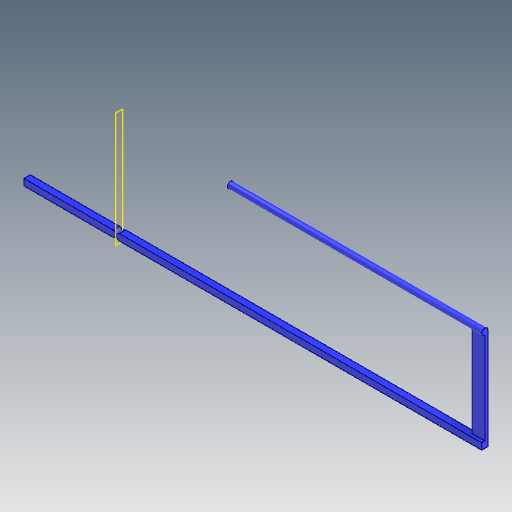
# Autodesk Inventor part: Bone_16_10_Fix
Saved by Autodesk Inventor 2020 (Build 240168000, 168)
## iProperties
Created: 2021-03-17
Part Number: Bone_16_10_Fix
Material: Generic
Document SubType Name: Modeling
Designer: deox
Density: 1 g/cm^3
Appearance: Blue - Wall Paint - Glossy
Author: deox
Autodesk Inventor part; units mm, degrees
ref_plane "YZ Plane" through (0, 0, 0) normal (1, 0, 0) x (0, 1, 0)
ref_plane "XZ Plane" through (0, 0, 0) normal (0, 1, 0) x (-1, 0, 0)
ref_plane "XY Plane" through (0, 0, 0) normal (0, 0, 1) x (1, 0, 0)
sketch "Sketch1" plane through (0, 0, 0) normal (1, 0, 0) x (0, 1, 0)
  circle A0 centre (0, 0) radius 0.05
  line L0 (0, 0) -> (-1.539, 0)
  line L1 (-1.589, 0.05) -> (-1.489, 0.05)
  line L2 (-1.489, 0.05) -> (-1.489, -0.05)
  line L3 (-1.489, -0.05) -> (-1.589, -0.05)
  line L4 (-1.589, -0.05) -> (-1.589, 0.05)
  line L5 (-1.589, 0.05) -> (-1.489, -0.05) construction
  line L6 (-1.489, 0.05) -> (-1.589, -0.05) construction
  line L7 (-1.489, -0.05) -> (0, -0.05)
  point P0 (-0.05, 0)
  point P1 (-1.489, 0)
  dimension "d0" = 0.1
  dimension "d1" = 1.539
  dimension "d2" = 0.1
  dimension "d3" = 0.1
  constraints: 16 end point, 2 horizontal, 2 midpoint, 2 parallel, 1 coincident, 1 perpendicular, 1 point on line, 3 other
  measures "d1" distance of L0.start L0.end
  measures "d2" distance of L2.end L3.end
  measures "d3" distance of L1.end L2.end
extrude "Extrusion1" add sketch "Sketch1" along normal blind 0.2
sketch "Sketch2" plane through (0, 0, 0) normal (-1, 0, 0) x (0, 0, 1)
  arc A0 (0, -0.05) -> (-0.05, 0) centre (0, 0) ccw projected
  circle A1 centre (0, 0) radius 0.05
  point P0 (-0.05, 0)
  point P1 (0, -0.05)
  dimension "d6" = 0.1
  constraints: 1 centre point, 1 coincident
  measures "d6" diameter of A1
extrude "Extrusion2" add sketch "Sketch2" along normal blind 3.8
sketch "Sketch3" plane through (0, 0, 0) normal (-1, 0, 0) x (0, 0, 1)
  line L0 (-0.05, -1.589) -> (-0.05, 0) projected
  line L1 (0.05, -1.589) -> (-0.05, -1.589) projected
  line L2 (-0.05, -1.589) -> (0.05, -1.589)
  line L3 (0, -1.489) -> (0.05, -1.489) projected
  line L4 (0.05, -1.589) -> (0.05, -1.489)
  line L5 (0.05, -1.489) -> (-0.05, -1.489)
  line L6 (-0.05, -1.489) -> (-0.05, -1.589)
  point P0 (0, 0)
  constraints: 8 end point, 3 perpendicular, 1 collinear, 1 point on line
extrude "Extrusion3" add sketch "Sketch3" along normal blind 7
ref_plane "Work Plane1" through (-5.55, 0, 0) normal (1, 0, 0) x (0, 0, -1)
split body "Split1" result two bodies by plane through (-5.55, 0, 0) normal (1, 0, 0) first body at (-1.2667, -0.0285, 0.0093)
sketch "Sketch5" plane through (-7, -1.589, -0.05) normal (0, 0, -1) x (-1, 0, 0)
  line L0 (-1.45, 0.1) -> (-1.45, 0) projected
  line L1 (-1.45, 0.05) -> (-1.4, 0.05)
  circle A0 centre (-1.4, 0.05) radius 0.05
  line L2 (-1.45, 0) -> (-7.2, 0) projected
  line L3 (-1.45, 0) -> (-1.45, 0.1)
  line L4 (-7, 0.1) -> (-1.45, 0.1) projected
  line L5 (-1.45, 0.1) -> (-1.4, 0.1)
  line L6 (-1.45, 0.1) -> (0, 0.1) projected
  line L7 (-1.45, 0) -> (-1.4, 0)
  line L8 (-1.45, 0) -> (0, 0) projected
  point P0 (-7, 1.589)
  dimension "d14" = 0.05
  constraints: 8 end point, 3 point on circle, 2 point on line, 1 centre point, 1 coincident, 1 horizontal, 1 midpoint, 1 perpendicular
  measures "d14" distance of L1.start L1.end
extrude "Extrusion5" cut sketch "Sketch5" against normal blind 10 contours L5 A0 L0 | A0 L7 L0 bodies 3
sketch "Sketch6" plane through (0, -1.489, -0.05) normal (0, 0, -1) x (-1, 0, 0)
  line L0 (5.55, 0) -> (5.55, -0.1) projected
  line L1 (5.55, -0.05) -> (5.5, -0.05)
  circle A0 centre (5.5, -0.05) radius 0.05
  line L2 (0, 0) -> (5.55, 0) projected
  line L3 (5.5, 0) -> (5.55, 0)
  line L4 (5.55, -0.1) -> (-0.2, -0.1) projected
  line L5 (5.55, 0) -> (5.55, -0.1)
  line L6 (5.55, -0.1) -> (5.5, -0.1)
  point P0 (0, 1.489)
  dimension "d17" = 0.05
  constraints: 8 end point, 3 point on circle, 2 point on line, 1 centre point, 1 coincident, 1 collinear, 1 horizontal, 1 midpoint, 1 perpendicular
  measures "d17" distance of L1.start L1.end
extrude "Extrusion6" cut sketch "Sketch6" against normal blind 10 contours L0 A0 L2 | L0 L4 A0 bodies 2
body "Solid2"
body "Solid3"
